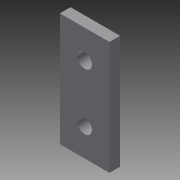
# Autodesk Inventor part: 4107
Saved by Autodesk Inventor 2014 SP2 (Build 180246200, 246)
## iProperties
Created: 2019-11-07
Part Number: 4107
Material: Generic
Catalog Web Link: www.cadenas.de
Description: 4107, 4307, 4107-Black, 4307-Black-Joining Plates - 2 Hole Joining Strip
Vendor: 8020
Document SubType Name: Modeling
Designer: psadmin
Manufacturer: 8020
Mass: 5.07172 g
Surface Area: 30.1746 cm^2
Volume: 5.07172 cm^3
Density: 1 g/cm^3
Appearance: PSOLRGB-191-191-191
Category: PARTsolutions
Company: 8020
Title: 4107
Author: Cadenas PARTsolutions
Comments: Joining Plates - 2 Hole Joining Strip
PSOL_IDENT_0: {$CADENAS_DATA\23d-libs\8020\inch\joining_plates\4107.prj},176 {VTYP=3D},{NB=4107},{LINA=4107},{NN=4
PSOL_IDENT_1: 107, 4307, 4107-Black, 4307-Black},{DATE=01.10.2019 06:04:23},{GEOMDATE=11.07.2017 14:05:39},{VERSIO
PSOL_IDENT_2: N=},{LINEID=10},{WBVAR=},{WBNUMERIC=}  {NB=4107},{LINA=4107},{KT=DUMMY},{PN=4107},{A=0.875},{B=2.000
PSOL_IDENT_3: },{F=0.257},{W=.030},{A1=0.4375},{C1=1.500},{C2=0.500},{D1=0.188},{COLOR=.75,.75,.75}
NN: 4107, 4307, 4107-Black, 4307-Black
NT: Joining Plates - 2 Hole Joining Strip
NB: 4107
NBSYN: $PN.
LINA: 4107
PN: 4107
A: 0.875
B: 2
W: .030
SUPPLIER: 8020
ARTICLENO: 4107
BOMINFO: 4107
CREATOR: CADENAS GmbH
Autodesk Inventor part; units mm, degrees
ref_plane "YZ Plane" through (0, 0, 0) normal (1, 0, 0) x (0, 1, 0)
ref_plane "XZ Plane" through (0, 0, 0) normal (0, 1, 0) x (-1, 0, 0)
ref_plane "XY Plane" through (0, 0, 0) normal (0, 0, 1) x (1, 0, 0)
sketch "Sketch_1" plane through (0, 0, 0) normal (0, 0, 1) x (1, 0, 0)
  line L0 (-11.1125, 50.8) -> (-11.1125, 0)
  line L1 (-11.1125, 0) -> (11.1125, 0)
  line L2 (11.1125, 0) -> (11.1125, 50.8)
  line L3 (11.1125, 50.8) -> (-11.1125, 50.8)
  circle A0 centre (0, 12.7) radius 3.2639
  circle A1 centre (0, 38.1) radius 3.2639
  constraints: 8 end point, 2 centre point
extrude "Extrusion1" add sketch "Sketch_1" along normal blind 4.7752
body "Solid1"
